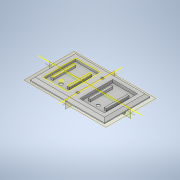
# Autodesk Inventor part: PV-Halterung
Saved by Autodesk Inventor 2021 (Build 250183000, 183)
## iProperties
Created: 2023-10-13
Part Number: PV-Halterung
Material: Generisch
Document SubType Name: Modeling
Designer: pasca
Density: 1 g/cm^3
Appearance: Vorgabe
Author: pasca
Autodesk Inventor part; units mm, degrees
sketch "Skizze1" plane through (0, 0, 0) normal (0, 0, 1) x (1, 0, 0)
  line L0 (0, 40) -> (0, -37) construction
  line L1 (-52, 0) -> (54, 0) construction
  line L2 (-90, -55) -> (90, -55)
  line L3 (90, -55) -> (90, 55)
  line L4 (90, 55) -> (-90, 55)
  line L5 (-90, 55) -> (-90, -55)
  line L6 (0, -77) -> (0, 77) projected
  line L7 (-126, 0) -> (126, 0) projected
  point P0 (0, 0)
  dimension "d0" = 110
  dimension "d1" = 180
  constraints: 12 end point, 2 horizontal, 2 parallel, 1 perpendicular, 1 vertical, 2 other
  measures "d0" distance between parallel lines of L2 L4
  measures "d1" distance between parallel lines of L3 L5
extrude "Extrusion1" add sketch "Skizze1" along normal blind 8
sketch "Skizze2" plane through (0, 0, 8) normal (0, 0, 1) x (1, 0, 0)
  line L0 (-75, 40) -> (-15, 40)
  line L1 (-15, 40) -> (-15, -40)
  line L2 (-15, -40) -> (-75, -40)
  line L3 (-75, -40) -> (-75, 40)
  line L4 (-126, 0) -> (126, 0) projected
  line L5 (0, 77) -> (0, -77) projected
  point P0 (0, 0)
  dimension "d4" = 60
  dimension "d5" = 80
  dimension "d6" = 15
  constraints: 8 end point, 2 parallel, 1 horizontal, 1 perpendicular, 1 other
  measures "d4" distance of L1.end L2.end
  measures "d5" distance of L0.end L1.end
  measures "d6" distance between parallel lines of L5 L1
extrude "Extrusion2" cut sketch "Skizze2" against normal blind 7
sketch "Skizze3" plane through (0, 0, 1) normal (0, 0, 1) x (1, 0, 0)
  line L0 (-15, 40) -> (-15, -40) projected
  line L1 (-15, -40) -> (-75, -40) projected
  line L2 (-75, -40) -> (-75, 40) projected
  line L3 (-15, -40) -> (-75, -40) projected
  line L4 (-15, 40) -> (-15, -40) projected
  line L5 (-75, 40) -> (-15, 40) projected
  line L6 (-126, 0) -> (126, 0) projected
  line L7 (0, 77) -> (0, -77) projected
  circle A0 centre (-45, -25) radius 4
  point P0 (0, 0)
  dimension "d9" = 8
  dimension "d10" = 30
  dimension "d11" = 15
  constraints: 1 centre point
  measures "d9" diameter of A0
  measures "d10" distance from line of L0 A0.centre
  measures "d11" distance from line of L1 A0.centre
extrude "Extrusion3" cut sketch "Skizze3" against normal blind 10 contours A0
sketch "Skizze4" plane through (0, 0, 1) normal (0, 0, 1) x (1, 0, 0)
  circle A0 centre (-45, -25) radius 4 projected
  line L0 (-75, -40) -> (-75, 40) projected
  line L1 (-15, -40) -> (-75, -40) projected
  line L2 (-15, 40) -> (-15, -40) projected
  line L3 (-75, 40) -> (-15, 40) projected
  line L4 (-126, 0) -> (126, 0) projected
  line L5 (-67, 27.5) -> (-62, 27.5)
  line L6 (-62, 27.5) -> (-62, -27.5)
  line L7 (-62, -27.5) -> (-67, -27.5)
  line L8 (-67, -27.5) -> (-67, 27.5)
  line L9 (-23, 27.5) -> (-28, 27.5)
  line L10 (-28, 27.5) -> (-28, -27.5)
  line L11 (-28, -27.5) -> (-23, -27.5)
  line L12 (-23, -27.5) -> (-23, 27.5)
  point P0 (0, 0)
  dimension "d14" = 5
  dimension "d15" = 55
  dimension "d16" = 8
  dimension "d17" = 55
  dimension "d18" = 5
  dimension "d19" = 8
  constraints: 16 end point, 4 parallel, 2 horizontal, 2 perpendicular, 2 other
  measures "d14" distance between parallel lines of L6 L8
  measures "d15" distance between parallel lines of L7 L5
  measures "d16" distance between parallel lines of L0 L8
  measures "d17" distance between parallel lines of L11 L9
  measures "d18" distance between parallel lines of L12 L10
  measures "d19" distance between parallel lines of L2 L12
extrude "Extrusion4" add sketch "Skizze4" along normal blind 5.5 contours L8 L5 L6 L4 | L4 L6 L7 L8 | L12 L11 L10 L4 | L4 L10 L9 L12
sketch "Skizze5" plane through (0, 0, 8) normal (0, 0, 1) x (1, 0, 0)
  line L0 (0, 77) -> (0, -77) projected
  line L1 (-126, 0) -> (126, 0) projected
  circle A0 centre (0, 30) radius 3
  circle A1 centre (0, -30) radius 3
  point P0 (0, 0)
  dimension "d22" = 6
  dimension "d23" = 6
  dimension "d24" = 30
  dimension "d25" = 30
  constraints: 2 centre point, 2 point on line
  measures "d22" diameter of A0
  measures "d23" diameter of A1
  measures "d24" distance of point (0, 0) A0.centre
  measures "d25" distance from line of L1 A1.centre
extrude "Extrusion5" cut sketch "Skizze5" against normal blind 10
sketch "Skizze6" plane through (0, 0, 8) normal (0, 0, 1) x (1, 0, 0)
  line L0 (-75, 40) -> (-15, 40) projected
  line L1 (-75, -40) -> (-75, 40) projected
  line L2 (-67, 27.5) -> (-67, -27.5) projected
  line L3 (-62, -27.5) -> (-62, 27.5) projected
  line L4 (-62, 27.5) -> (-67, 27.5) projected
  line L5 (-67, -27.5) -> (-62, -27.5) projected
  line L6 (-15, -40) -> (-75, -40) projected
  circle A0 centre (-45, -25) radius 4 projected
  line L7 (-28, 27.5) -> (-28, -27.5) projected
  line L8 (-28, -27.5) -> (-23, -27.5) projected
  line L9 (-23, -27.5) -> (-23, 27.5) projected
  line L10 (-23, 27.5) -> (-28, 27.5) projected
  line L11 (-28, 27.5) -> (-28, -27.5) projected
  line L12 (-28, -27.5) -> (-23, -27.5) projected
  line L13 (-15, 40) -> (-15, -40) projected
  line L14 (0, 77) -> (0, -77) projected
  line L15 (-126, 0) -> (126, 0) projected
  point P0 (0, 0)
mirror "Spiegeln1" about plane through (0, 0, 0) normal (1, 0, 0) of "Extrusion4", "Extrusion2", "Extrusion3"
sketch "Skizze7" plane through (0, 0, 0) normal (0, 0, -1) x (-1, 0, 0)
  point P0 (0, 0)
sketch "Skizze8" plane through (0, 0, 0) normal (1, 0, 0) x (0, 1, 0)
  circle A0 centre (0, -7) radius 1.65
  circle A1 centre (0, -7) radius 4
  line L0 (55, 0) -> (-55, 0) projected
  line L1 (4, 0) -> (4, -7)
  line L2 (-4, -7) -> (-4, 0)
  point P0 (0, 0)
  dimension "d28" = 3.3
  dimension "d29" = 7
  dimension "d30" = 8
  constraints: 4 end point, 2 centre point, 2 point on circle, 2 point on line, 1 coincident, 1 parallel, 1 tangent
  measures "d28" diameter of A0
  measures "d29" distance of A0.centre point (0, 0)
  measures "d30" diameter of A1
extrude "Extrusion6" add sketch "Skizze8" along normal mid plane 6
pattern_linear "Rechteckige Anordnung1" count 2 spacing 80 along (-1, 0, 0) of "Extrusion6"
pattern_linear "Rechteckige Anordnung2" count 2 spacing 80 along (1, 0, 0) of "Extrusion6"
chamfer "Fase1" distance 6 angle 45 4 edges at (0, 55, 8) (-90, 0, 8) (0, -55, 8) (90, 0, 8)
